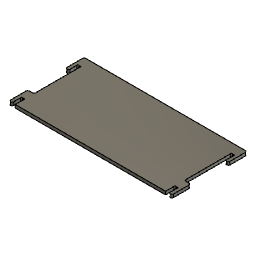
Lid_Base_Cut2 (Autodesk Fusion 360 design; units mm, degrees)
Autodesk Fusion 360 part; units mm, degrees
sketch "Sketch1" plane through (0, 0, 0) normal (0, 1, 0) x (1, 0, 0)
  line L0 (0, 0) -> (609.6, 0)
  line L1 (609.6, 0) -> (609.6, -304.8)
  line L2 (609.6, -304.8) -> (0, -304.8)
  line L3 (0, -304.8) -> (0, 0)
  line L4 (0, 0) -> (-25.4, 0)
  line L5 (-25.4, 0) -> (-25.4, -76.2)
  line L6 (-25.4, -76.2) -> (-12.7, -76.2)
  line L7 (-12.7, -76.2) -> (-12.7, -38.1)
  line L8 (-12.7, -38.1) -> (0, -38.1)
  line L9 (0, -304.8) -> (0, -228.6) construction
  line L10 (0, -228.6) -> (-25.4, -228.6)
  line L11 (-25.4, -228.6) -> (-25.4, -304.8)
  line L12 (-25.4, -304.8) -> (-12.7, -304.8)
  line L13 (-12.7, -304.8) -> (-12.7, -266.7)
  line L14 (-12.7, -266.7) -> (0, -266.7)
  line L15 (609.6, 0) -> (635, 0)
  line L16 (635, 0) -> (635, -76.2)
  line L17 (635, -76.2) -> (622.3, -76.2)
  line L18 (622.3, -76.2) -> (622.3, -38.1)
  line L19 (622.3, -38.1) -> (609.6, -38.1)
  line L20 (609.6, -304.8) -> (609.6, -228.6) construction
  line L21 (609.6, -228.6) -> (635, -228.6)
  line L22 (635, -228.6) -> (635, -304.8)
  line L23 (635, -304.8) -> (622.3, -304.8)
  line L24 (622.3, -304.8) -> (622.3, -266.7)
  line L25 (622.3, -266.7) -> (609.6, -266.7)
  dimension "d1" = 609.6
  dimension "d2" = 304.8
  dimension "d3" = 25.4
  dimension "d4" = 76.2
  dimension "d5" = 38.1
  dimension "d6" = 76.2
  dimension "d7" = 25.4
  dimension "d8" = 76.2
  dimension "d9" = 38.1
  dimension "d10" = 25.4
  dimension "d11" = 76.2
  dimension "d12" = 76.2
  dimension "d13" = 25.4
  dimension "d14" = 38.1
  constraint horizontal L0
  constraint vertical L1
  constraint horizontal L2
  constraint vertical L3
  constraint coincident L0.start L3.end
  constraint horizontal L4
  constraint perpendicular L4 L5
  constraint perpendicular L5 L6
  constraint perpendicular L6 L7
  constraint coincident L3 L8.end
  constraint perpendicular L3 L8
  constraint perpendicular L2 L9
  constraint perpendicular L9 L10
  constraint perpendicular L10 L11
  constraint perpendicular L11 L12
  constraint perpendicular L12 L13
  constraint midpoint L9 L14.end
  constraint perpendicular L1 L15
  constraint perpendicular L15 L16
  constraint perpendicular L16 L17
  constraint perpendicular L17 L18
  constraint coincident L1 L19.end
  constraint perpendicular L1 L19
  constraint perpendicular L2 L20
  constraint perpendicular L20 L21
  constraint perpendicular L21 L22
  constraint perpendicular L22 L23
  constraint perpendicular L21 L24
  constraint midpoint L20 L25.end
  measures "d1" distance of L0.start L0.end
  measures "d2" distance of L0.start L2.end
  measures "d3" distance of L0.start L4.end
  measures "d4" distance of L4.end L5.end
  measures "d5" distance of L6.end L7.end
  measures "d6" distance of L2.end L9.end
  measures "d7" distance of L9.end L10.end
  measures "d8" distance of L10.end L11.end
  measures "d9" distance of L12.end L13.end
  measures "d10" distance of L0.end L15.end
  measures "d11" distance of L15.end L16.end
  measures "d12" distance of L1.end L20.end
  measures "d13" distance of L20.end L21.end
  measures "d14" distance of L23.end L24.end
extrude "Extrude1" add sketch "Sketch1" along normal blind 12.7 in component "Component"
fillet "Fillet1" radius 6.35 14 edges at (-25.4, 6.35, 0) (-25.4, 6.35, 228.6) (-25.4, 6.35, 76.2) (-12.7, 6.35, 76.2) (-25.4, 6.35, 304.8) (-12.7, 6.35, 304.8) (635, 6.35, 304.8) (622.3, 6.35, 304.8) (635, 6.35, 228.6) (609.6, 6.35, 228.6) (0, 6.35, 228.6) (635, 6.35, 76.2) (622.3, 6.35, 76.2) (635, 6.35, 0) in component "Component"
ref_plane "WorkPlane1" through (-12.7, 0, 38.1) normal (0, 1, 0) x (-1, 0, 0)
sketch "Sketch2" plane through (-12.7, 0, 38.1) normal (0, 1, 0) x (-1, 0, 0)
  line L0 (0, 31.75) -> (0, 0) construction
  line L1 (0, 0) -> (-12.7, 0) construction
  line L2 (0, 0) -> (-2.2451, 2.2451) construction
  circle A0 centre (-2.2451, 2.2451) radius 3.175
  dimension "d20" = 3.175
  constraint coincident L0.end L1.start
  constraint coincident L0.end A0
  measures "d20" distance of L0.end L2.end
sweep "Sweep1" cut kept parallel profiles "Sketch2" along 1 edges at (-12.7, 6.35, 38.1) section 1 in component "Component"
ref_plane "WorkPlane2" through (0, 0, 38.1) normal (0, 1, 0) x (-1, 0, 0)
sketch "Sketch3" plane through (0, 0, 38.1) normal (0, 1, 0) x (-1, 0, 0)
  line L0 (8.2099, 0) -> (0, 0) construction
  line L1 (0, 184.15) -> (0, 0) construction
  line L2 (0, 0) -> (2.2451, 2.2451) construction
  circle A0 centre (2.2451, 2.2451) radius 3.175
  dimension "d28" = 3.175
  constraint coincident L0.end L1.end
  constraint coincident L0.end A0
  measures "d28" distance of L0.end L2.end
sweep "Sweep2" cut kept parallel profiles "Sketch3" along 1 edges at (0, 6.35, 38.1) section 1 in component "Component"
ref_plane "WorkPlane3" through (0, 0, 266.7) normal (0, 1, 0) x (-1, 0, 0)
sketch "Sketch4" plane through (0, 0, 266.7) normal (0, 1, 0) x (-1, 0, 0)
  line L0 (12.7, 0) -> (0, 0) construction
  line L1 (0, 38.1) -> (0, 0) construction
  line L2 (0, 0) -> (2.2451, 2.2451) construction
  circle A0 centre (2.2451, 2.2451) radius 3.175
  dimension "d36" = 3.175
  constraint coincident L0.end L1.end
  constraint coincident L0.end A0
  measures "d36" distance of L0.end L2.end
sweep "Sweep3" cut kept parallel profiles "Sketch4" along 1 edges at (0, 6.35, 266.7) section 1 in component "Component"
ref_plane "WorkPlane4" through (-12.7, 0, 266.7) normal (0, 1, 0) x (-1, 0, 0)
sketch "Sketch5" plane through (-12.7, 0, 266.7) normal (0, 1, 0) x (-1, 0, 0)
  line L0 (0, 31.75) -> (0, 0) construction
  line L1 (0, 0) -> (-8.2099, 0) construction
  line L2 (0, 0) -> (-2.2451, 2.2451) construction
  circle A0 centre (-2.2451, 2.2451) radius 3.175
  dimension "d44" = 3.175
  constraint coincident L0.end L1.start
  constraint coincident L0.end A0
  measures "d44" distance of L0.end L2.end
sweep "Sweep4" cut kept parallel profiles "Sketch5" along 1 edges at (-12.7, 6.35, 266.7) section 1 in component "Component"
ref_plane "WorkPlane5" through (622.3, 0, 38.1) normal (0, 1, 0) x (-1, 0, 0)
sketch "Sketch6" plane through (622.3, 0, 38.1) normal (0, 1, 0) x (-1, 0, 0)
  line L0 (0, 0) -> (12.7, 0) construction
  line L1 (0, 31.75) -> (0, 0) construction
  line L2 (0, 0) -> (2.2451, 2.2451) construction
  circle A0 centre (2.2451, 2.2451) radius 3.175
  dimension "d52" = 3.175
  constraint coincident L0.start L1.end
  constraint coincident L0.start A0
  measures "d52" distance of L0.start L2.end
sweep "Sweep5" cut kept parallel profiles "Sketch6" along 1 edges at (622.3, 6.35, 38.1) section 1 in component "Component"
ref_plane "WorkPlane6" through (609.6, 0, 38.1) normal (0, 1, 0) x (-1, 0, 0)
sketch "Sketch7" plane through (609.6, 0, 38.1) normal (0, 1, 0) x (-1, 0, 0)
  line L0 (0, 0) -> (0, 184.15) construction
  line L1 (-8.2099, 0) -> (0, 0) construction
  line L2 (0, 0) -> (-2.2451, 2.2451) construction
  circle A0 centre (-2.2451, 2.2451) radius 3.175
  dimension "d60" = 3.175
  constraint coincident L0.start L1.end
  constraint coincident L0.start A0
  measures "d60" distance of L0.start L2.end
sweep "Sweep6" cut kept parallel profiles "Sketch7" along 1 edges at (609.6, 6.35, 38.1) section 1 in component "Component"
ref_plane "WorkPlane7" through (609.6, 0, 266.7) normal (0, 1, 0) x (-1, 0, 0)
sketch "Sketch8" plane through (609.6, 0, 266.7) normal (0, 1, 0) x (-1, 0, 0)
  line L0 (0, 0) -> (0, 38.1) construction
  line L1 (-12.7, 0) -> (0, 0) construction
  line L2 (0, 0) -> (-2.2451, 2.2451) construction
  circle A0 centre (-2.2451, 2.2451) radius 3.175
  dimension "d68" = 3.175
  constraint coincident L0.start L1.end
  constraint coincident L0.start A0
  measures "d68" distance of L0.start L2.end
sweep "Sweep7" cut kept parallel profiles "Sketch8" along 1 edges at (609.6, 6.35, 266.7) section 1 in component "Component"
ref_plane "WorkPlane8" through (622.3, 0, 266.7) normal (0, 1, 0) x (-1, 0, 0)
sketch "Sketch9" plane through (622.3, 0, 266.7) normal (0, 1, 0) x (-1, 0, 0)
  line L0 (0, 0) -> (8.2099, 0) construction
  line L1 (0, 31.75) -> (0, 0) construction
  line L2 (0, 0) -> (2.2451, 2.2451) construction
  circle A0 centre (2.2451, 2.2451) radius 3.175
  dimension "d76" = 3.175
  constraint coincident L0.start L1.end
  constraint coincident L0.start A0
  measures "d76" distance of L0.start L2.end
sweep "Sweep8" cut kept parallel profiles "Sketch9" along 1 edges at (622.3, 6.35, 266.7) section 1 in component "Component"
component "Component" placed x (1, 0, 0) y (0, 1, 0) z (0, 0, 1) at (0, 0, 0)
equation "d20 = 0.25 in / 2 + 0.00 in"
equation "d28 = 0.25 in / 2 + 0.00 in"
equation "d36 = 0.25 in / 2 + 0.00 in"
equation "d44 = 0.25 in / 2 + 0.00 in"
equation "d52 = 0.25 in / 2 + 0.00 in"
equation "d60 = 0.25 in / 2 + 0.00 in"
equation "d68 = 0.25 in / 2 + 0.00 in"
equation "d76 = 0.25 in / 2 + 0.00 in"
